Autodesk Inventor part; units mm, degrees
(part 2 of 2)
sketch "Sketch18" plane through (0, 3, 0) normal (0, 1, 0) x (1, 0, 0)
  line L0 (-26.0093, -14.7158) -> (-51.6764, -14.7158)
  line L1 (-51.6764, -14.7158) -> (-51.6764, 17.4536)
  line L2 (-51.6764, 17.4536) -> (-26.0093, 17.4536)
  line L3 (-26.0093, 17.4536) -> (-26.0093, -14.7158)
  line L4 (-61.1366, 28.9911) -> (-74.2787, 28.9911)
  line L5 (-74.2787, 28.9911) -> (-74.2787, 55.1603)
  line L6 (-74.2787, 55.1603) -> (-61.1366, 55.1603)
  line L7 (-61.1366, 55.1603) -> (-61.1366, 28.9911)
  line L8 (-71.136, 57.3703) -> (-87.7064, 57.3703)
  line L9 (-87.7064, 57.3703) -> (-87.7064, 38.1334)
  line L10 (-87.7064, 38.1334) -> (-71.136, 38.1334)
  line L11 (-71.136, 38.1334) -> (-71.136, 57.3703)
  line L12 (-73.3824, 30.8203) -> (-76.7813, 30.8203)
  line L13 (-76.7813, 30.8203) -> (-76.7813, 40.4219)
  line L14 (-76.7813, 40.4219) -> (-73.3824, 40.4219)
  line L15 (-73.3824, 40.4219) -> (-73.3824, 30.8203)
  line L16 (-76.3763, 32.094) -> (-79.4212, 32.094)
  line L17 (-79.4212, 32.094) -> (-79.4212, 39.2374)
  line L18 (-79.4212, 39.2374) -> (-76.3763, 39.2374)
  line L19 (-76.3763, 39.2374) -> (-76.3763, 32.094)
  line L20 (-79.1582, 33.8973) -> (-82.4713, 33.8973)
  line L21 (-82.4713, 33.8973) -> (-82.4713, 38.9159)
  line L22 (-82.4713, 38.9159) -> (-79.1582, 38.9159)
  line L23 (-79.1582, 38.9159) -> (-79.1582, 33.8973)
  line L24 (-82.2476, 35.5049) -> (-85.0994, 35.5049)
  line L25 (-85.0994, 35.5049) -> (-85.0994, 38.3288)
  line L26 (-85.0994, 38.3288) -> (-82.2476, 38.3288)
  line L27 (-82.2476, 38.3288) -> (-82.2476, 35.5049)
  line L28 (-84.8897, 37.1825) -> (-86.2724, 37.1825)
  line L29 (-86.2724, 37.1825) -> (-86.2724, 39.3493)
  line L30 (-86.2724, 39.3493) -> (-84.8897, 39.3493)
  line L31 (-84.8897, 39.3493) -> (-84.8897, 37.1825)
  point P0 (0, 0)
  constraints: 64 end point, 16 parallel, 8 horizontal, 8 perpendicular
extrude "Extrusion18" add sketch "Sketch18" against normal blind 3 contours L4 L5 L12 L15 L10 L11 L6 L7 | L12 L13 L16 L19 L10 L5 | L5 L10 L15 L12 | L11 L10 L15 L14 L5 L6 | L6 L5 L14 L13 L18 L17 L22 L21 L26 L31 L30 L29 L10 L9 L8 L11 | L10 L19 L18 L13 L14 L5 | L5 L14 L15 L10 | L19 L16 L13 L10 | L10 L13 L18 L19 | L16 L17 L20 L23 L10 L13 | L10 L23 L22 L17 L18 L13 | L23 L20 L17 L10 | L10 L17 L22 L23 | L20 L21 L24 L27 L10 L17 | L29 L30 L31 L26 L25 L10 | L10 L27 L26 L21 L22 L17 | L25 L26 L31 L10 | L10 L31 L28 L25 | L27 L24 L21 L10 | L10 L21 L26 L27 | L24 L25 L28 L31 L10 L21 | L31 L26 L21 L10
sketch "Sketch19" plane through (0, 3, 0) normal (0, 1, 0) x (1, 0, 0)
  line L0 (-25.8067, -16.6131) -> (-52.5812, -16.6131)
  line L1 (-52.5812, -16.6131) -> (-52.5812, 17.0969)
  line L2 (-52.5812, 17.0969) -> (-25.8067, 17.0969)
  line L3 (-25.8067, 17.0969) -> (-25.8067, -16.6131)
  line L4 (33.7548, 15.1527) -> (6.613, 15.1527)
  line L5 (6.613, 15.1527) -> (6.613, 48.065)
  line L6 (6.613, 48.065) -> (33.7548, 48.065)
  line L7 (33.7548, 48.065) -> (33.7548, 15.1527)
  line L8 (13.7098, 76.1298) -> (-12.5808, 76.1298)
  line L9 (-12.5808, 76.1298) -> (-12.5808, 99.3558)
  line L10 (-12.5808, 99.3558) -> (13.7098, 99.3558)
  line L11 (13.7098, 99.3558) -> (13.7098, 76.1298)
  line L12 (36.1294, -49.0327) -> (2.2581, -49.0327)
  line L13 (2.2581, -49.0327) -> (2.2581, -15.484)
  line L14 (2.2581, -15.484) -> (36.1294, -15.484)
  line L15 (36.1294, -15.484) -> (36.1294, -49.0327)
  line L16 (13.7098, -98.7106) -> (-12.5808, -98.7106)
  line L17 (-12.5808, -98.7106) -> (-12.5808, -73.7104)
  line L18 (-12.5808, -73.7104) -> (13.7098, -73.7104)
  line L19 (13.7098, -73.7104) -> (13.7098, -98.7106)
  line L20 (86.7795, -30.086) -> (63.0132, -30.086)
  line L21 (63.0132, -30.086) -> (63.0132, -58.4963)
  line L22 (63.0132, -58.4963) -> (86.7795, -58.4963)
  line L23 (86.7795, -58.4963) -> (86.7795, -30.086)
  line L24 (90.7338, 30.2618) -> (63.0132, 30.2618)
  line L25 (63.0132, 30.2618) -> (63.0132, 42.7998)
  line L26 (63.0132, 42.7998) -> (90.7338, 42.7998)
  line L27 (90.7338, 42.7998) -> (90.7338, 30.2618)
  line L28 (87.513, 41.3045) -> (60.8267, 41.3045)
  line L29 (60.8267, 41.3045) -> (60.8267, 56.258)
  line L30 (60.8267, 56.258) -> (87.513, 56.258)
  line L31 (87.513, 56.258) -> (87.513, 41.3045)
  point P0 (0, 0)
  constraints: 64 end point, 16 parallel, 8 horizontal, 8 perpendicular, 3 point on line
extrude "Extrusion19" add sketch "Sketch19" against normal blind 3
sketch "Sketch20" plane through (0, 3, 0) normal (0, 1, 0) x (1, 0, 0)
  line L0 (-88.182, -39.8912) -> (-85.4044, -36.6086)
  line L1 (-85.4044, -36.6086) -> (-74.6729, -30.1276)
  line L2 (-74.6729, -30.1276) -> (-71.0115, -29.5805)
  line L3 (-71.0115, -29.5805) -> (-68.3289, -34.0226)
  line L4 (-68.3289, -34.0226) -> (-62.9313, -48.4344)
  line L5 (-62.9313, -48.4344) -> (-68.3289, -53.8736)
  line L6 (-68.3289, -53.8736) -> (-79.5547, -57.3142)
  line L7 (-79.5547, -57.3142) -> (-88.182, -39.8912)
  point P0 (0, 0)
  constraints: 16 end point, 1 perpendicular, 1 point on line
extrude "Extrusion20" add sketch "Sketch20" against normal blind 3
sketch "Sketch21" plane through (0, 3, 0) normal (0, 1, 0) x (1, 0, 0)
  line L0 (0, 0) -> (-34, 0)
  line L1 (-34, 0) -> (-26, 0)
  line L2 (-26, 0) -> (-26, 10)
  line L3 (-26, 10) -> (-42, 10)
  line L4 (-42, 10) -> (-42, -10)
  line L5 (-42, -10) -> (-26, -10)
  line L6 (-26, -10) -> (-26, 0)
  line L7 (0, 0) -> (17, 29.4449)
  line L8 (0, 0) -> (34, 0) construction
  line L9 (17, 29.4449) -> (13, 22.5167)
  line L10 (13, 22.5167) -> (4.3397, 27.5167)
  line L11 (4.3397, 27.5167) -> (12.3397, 41.3731)
  line L12 (12.3397, 41.3731) -> (29.6603, 31.3731)
  line L13 (29.6603, 31.3731) -> (21.6603, 17.5167)
  line L14 (21.6603, 17.5167) -> (13, 22.5167)
  line L15 (0, 0) -> (17, -29.4449)
  line L16 (0, 0) -> (34, 0) construction
  line L17 (17, -29.4449) -> (13, -22.5167)
  line L18 (13, -22.5167) -> (21.6603, -17.5167)
  line L19 (21.6603, -17.5167) -> (29.6603, -31.3731)
  line L20 (29.6603, -31.3731) -> (12.3397, -41.3731)
  line L21 (12.3397, -41.3731) -> (4.3397, -27.5167)
  line L22 (4.3397, -27.5167) -> (13, -22.5167)
  dimension "d187" = 34
  dimension "d188" = 8
  dimension "d189" = 10
  dimension "d190" = 16
  dimension "d191" = 20
  dimension "d192" = 34
  dimension "d193" = 60
  dimension "d194" = 8
  dimension "d195" = 10
  dimension "d196" = 16
  dimension "d197" = 20
  dimension "d198" = 16
  dimension "d199" = 34
  dimension "d200" = 60
  dimension "d201" = 10
  dimension "d202" = 16
  dimension "d203" = 20
  constraints: 46 end point, 13 perpendicular, 6 point on line, 3 horizontal, 2 equal length
  measures "d187" distance of L0.start L0.end
  measures "d188" distance of L0.end L1.end
  measures "d189" distance of L1.end L2.end
  measures "d190" distance of L2.end L3.end
  measures "d191" distance of L3.end L4.end
  measures "d192" distance of L0.start L7.end
  measures "d193" angle of L8 L7
  measures "d194" distance of L7.end L9.end
  measures "d195" distance of L9.end L10.end
  measures "d196" distance of L10.end L11.end
  measures "d197" distance of L11.end L12.end
  measures "d198" distance of L12.end L13.end
  measures "d199" distance of L0.start L15.end
  measures "d200" angle of L15 L16
  measures "d201" distance of L17.end L18.end
  measures "d202" distance of L18.end L19.end
  measures "d203" distance of L19.end L20.end
extrude "Extrusion21" cut sketch "Sketch21" against normal blind 3
sketch "Sketch22" plane through (0, 3, 0) normal (0, 1, 0) x (1, 0, 0)
  line L0 (0, 0) -> (-73.6122, -42.5)
  line L1 (0, 0) -> (85, 0) construction
  line L2 (-73.6122, -42.5) -> (-64.9519, -37.5)
  line L3 (-64.9519, -37.5) -> (-68.9519, -30.5718)
  line L4 (-68.9519, -30.5718) -> (-86.2724, -40.5718)
  line L5 (-86.2724, -40.5718) -> (-78.2724, -54.4282)
  line L6 (-78.2724, -54.4282) -> (-60.9519, -44.4282)
  line L7 (-60.9519, -44.4282) -> (-64.9519, -37.5)
  line L8 (0, 0) -> (-73.6122, 42.5)
  line L9 (0, 0) -> (85, 0) construction
  line L10 (-73.6122, 42.5) -> (-64.9519, 37.5)
  line L11 (-64.9519, 37.5) -> (-68.9519, 30.5718)
  line L12 (-68.9519, 30.5718) -> (-86.2724, 40.5718)
  line L13 (-86.2724, 40.5718) -> (-78.2724, 54.4282)
  line L14 (-78.2724, 54.4282) -> (-60.9519, 44.4282)
  line L15 (-60.9519, 44.4282) -> (-64.9519, 37.5)
  line L16 (0, 0) -> (0, 85)
  line L17 (0, 85) -> (0, 75)
  line L18 (0, 75) -> (-8, 75)
  line L19 (-8, 75) -> (-8, 95)
  line L20 (-8, 95) -> (8, 95)
  line L21 (8, 95) -> (8, 75)
  line L22 (8, 75) -> (0, 75)
  line L23 (0, 0) -> (73.6122, 42.5)
  line L24 (0, 0) -> (85, 0) construction
  line L25 (73.6122, 42.5) -> (64.9519, 37.5)
  line L26 (64.9519, 37.5) -> (60.9519, 44.4282)
  line L27 (60.9519, 44.4282) -> (78.2724, 54.4282)
  line L28 (78.2724, 54.4282) -> (86.2724, 40.5718)
  line L29 (86.2724, 40.5718) -> (68.9519, 30.5718)
  line L30 (64.9519, 37.5) -> (68.9519, 30.5718)
  line L31 (0, 0) -> (73.6122, -42.5)
  line L32 (73.6122, -42.5) -> (77.6122, -35.5718)
  line L33 (77.6122, -35.5718) -> (68.9519, -30.5718)
  line L34 (68.9519, -30.5718) -> (60.9519, -44.4282)
  line L35 (60.9519, -44.4282) -> (78.2724, -54.4282)
  line L36 (78.2724, -54.4282) -> (86.2724, -40.5718)
  line L37 (86.2724, -40.5718) -> (77.6122, -35.5718)
  line L38 (0, 0) -> (0, -85)
  line L39 (0, -85) -> (0, -75)
  line L40 (0, -75) -> (8, -75)
  line L41 (8, -75) -> (8, -95)
  line L42 (8, -95) -> (-8, -95)
  line L43 (-8, -95) -> (-8, -75)
  line L44 (0, -75) -> (-8, -75)
  dimension "d206" = 85
  dimension "d207" = 150
  dimension "d208" = 10
  dimension "d209" = 8
  dimension "d210" = 20
  dimension "d211" = 16
  dimension "d212" = 85
  dimension "d213" = 150
  dimension "d214" = 8
  dimension "d215" = 20
  dimension "d216" = 16
  dimension "d217" = 85
  dimension "d218" = 10
  dimension "d219" = 8
  dimension "d220" = 20
  dimension "d221" = 16
  dimension "d222" = 85
  dimension "d223" = 30
  dimension "d224" = 8
  dimension "d225" = 20
  dimension "d226" = 20
  dimension "d227" = 10
  dimension "d228" = 20
  dimension "d229" = 16
  constraints: 90 end point, 25 point on line, 23 perpendicular, 3 equal length, 3 horizontal, 1 vertical
  measures "d206" distance of L0.start L0.end
  measures "d207" angle of L0 L1
  measures "d208" distance of L0.end L2.end
  measures "d209" distance of L2.end L3.end
  measures "d210" distance of L3.end L4.end
  measures "d211" distance of L4.end L5.end
  measures "d212" distance of L0.start L8.end
  measures "d213" angle of L9 L8
  measures "d214" distance of L10.end L11.end
  measures "d215" distance of L11.end L12.end
  measures "d216" distance of L12.end L13.end
  measures "d217" distance of L0.start L16.end
  measures "d218" distance of L16.end L17.end
  measures "d219" distance of L17.end L18.end
  measures "d220" distance of L18.end L19.end
  measures "d221" distance of L19.end L20.end
  measures "d222" distance of L0.start L23.end
  measures "d223" angle of L24 L23
  measures "d224" distance of L25.end L26.end
  measures "d225" distance of L26.end L27.end
  measures "d226" distance of L34.end L35.end
  measures "d227" distance of L38.end L39.end
  measures "d228" distance of L40.end L41.end
  measures "d229" distance of L41.end L42.end
extrude "Extrusion22" cut sketch "Sketch22" against normal blind 3
sketch "Sketch23" plane through (0, 3, 0) normal (0, 1, 0) x (1, 0, 0)
  point P0 (0, 0)
fillet "Fillet11" radius 2 12 edges at (-8, 1.5, -95) (8, 1.5, -95) (8, 1.5, -75) (-8, 1.5, -75) (-78.2724, 1.5, -54.4282) (-86.2724, 1.5, -40.5718) (-60.9519, 1.5, -44.4282) (-68.9519, 1.5, -30.5718) (-26, 1.5, -10) (-42, 1.5, -10) (-42, 1.5, 10) (-26, 1.5, 10)
fillet "Fillet12" radius 2 12 edges at (4.3397, 1.5, -27.5167) (12.3397, 1.5, -41.3731) (29.6603, 1.5, -31.3731) (21.6603, 1.5, -17.5167) (60.9519, 1.5, -44.4282) (78.2724, 1.5, -54.4282) (86.2724, 1.5, -40.5718) (68.9519, 1.5, -30.5718) (60.9519, 1.5, 44.4282) (68.9519, 1.5, 30.5718) (86.2724, 1.5, 40.5718) (78.2724, 1.5, 54.4282)
fillet "Fillet13" radius 2 8 edges at (29.6603, 1.5, 31.3731) (21.6603, 1.5, 17.5167) (4.3397, 1.5, 27.5167) (12.3397, 1.5, 41.3731) (-8, 1.5, 75) (8, 1.5, 75) (8, 1.5, 95) (-8, 1.5, 95)
fillet "Fillet14" radius 2 4 edges at (-68.9519, 1.5, 30.5718) (-60.9519, 1.5, 44.4282) (-78.2724, 1.5, 54.4282) (-86.2724, 1.5, 40.5718)
sketch "Sketch24" plane through (0, 3, 0) normal (0, 1, 0) x (1, 0, 0)
  line L0 (0, 0) -> (22.5, 38.9711)
  line L1 (14.0718, 40.3731) -> (27.9282, 32.3731) projected
  line L2 (0, 0) -> (45, 0) construction
  line L3 (0, 0) -> (22.5, -38.9711)
  line L4 (14.0718, -40.3731) -> (27.9282, -32.3731) projected
  line L5 (0, 0) -> (45, 0) construction
  line L6 (0, 0) -> (-45, 0)
  circle A0 centre (22.5, 38.9711) radius 1.5
  circle A1 centre (22.5, -38.9711) radius 1.5
  circle A2 centre (-45, 0) radius 1.5
  dimension "d236" = 45
  dimension "d237" = 60
  dimension "d238" = 45
  dimension "d239" = 60
  dimension "d240" = 45
  dimension "d241" = 3
  dimension "d242" = 3
  constraints: 10 end point, 3 centre point, 3 coincident, 3 horizontal, 2 equal length, 2 perpendicular
  measures "d236" distance of L0.start L0.end
  measures "d237" angle of L2 L0
  measures "d238" distance of L0.start L3.end
  measures "d239" angle of L3 L5
  measures "d240" distance of L0.start L6.end
  measures "d241" diameter of A0
  measures "d242" diameter of A2
extrude "Extrusion23" cut sketch "Sketch24" against normal blind 3
sketch "Sketch25" plane through (0, 3, 0) normal (0, 1, 0) x (1, 0, 0)
  line L0 (-85.2724, -42.3038) -> (-79.2724, -52.6962) projected
  line L1 (-82.2724, -47.5) -> (-80.7724, -50.0981)
  line L2 (-82.2724, -47.5) -> (-84.8705, -49)
  circle A0 centre (-84.8705, -49) radius 1.5
  line L3 (-61.9519, -42.6962) -> (-67.9519, -32.3038) projected
  line L4 (-64.9519, -37.5) -> (-66.4519, -34.9019)
  line L5 (-66.4519, -34.9019) -> (-64.9519, -37.5)
  line L6 (-64.9519, -37.5) -> (-62.3538, -36)
  circle A1 centre (-62.3538, -36) radius 1.5
  line L7 (-67.9519, 32.3038) -> (-61.9519, 42.6962) projected
  line L8 (-64.9519, 37.5) -> (-63.4519, 40.0981)
  line L9 (-63.4519, 40.0981) -> (-64.9519, 37.5)
  line L10 (-64.9519, 37.5) -> (-62.3538, 36)
  circle A2 centre (-62.3538, 36) radius 1.5
  line L11 (-79.2724, 52.6962) -> (-85.2724, 42.3038) projected
  line L12 (-82.2724, 47.5) -> (-83.7724, 44.9019)
  line L13 (-83.7724, 44.9019) -> (-82.2724, 47.5)
  line L14 (-82.2724, 47.5) -> (-84.8705, 49)
  circle A3 centre (-84.8705, 49) radius 1.5
  line L15 (6, 95) -> (-6, 95) projected
  line L16 (0, 95) -> (0, 98)
  line L17 (-6, 75) -> (6, 75) projected
  line L18 (0, 75) -> (0, 72)
  circle A4 centre (0, 72) radius 1.5
  circle A5 centre (0, 98) radius 1.5
  line L19 (79.2724, 52.6962) -> (85.2724, 42.3038) projected
  line L20 (82.2724, 47.5) -> (83.7724, 44.9019)
  line L21 (83.7724, 44.9019) -> (82.2724, 47.5)
  line L22 (82.2724, 47.5) -> (84.8705, 49)
  line L23 (67.9519, 32.3038) -> (61.9519, 42.6962) projected
  line L24 (64.9519, 37.5) -> (63.4519, 40.0981)
  line L25 (63.4519, 40.0981) -> (64.9519, 37.5)
  line L26 (64.9519, 37.5) -> (62.3538, 36)
  circle A6 centre (62.3538, 36) radius 1.5
  circle A7 centre (84.8705, 49) radius 1.5
  line L27 (85.2724, -42.3038) -> (79.2724, -52.6962) projected
  line L28 (82.2724, -47.5) -> (80.7724, -50.0981)
  line L29 (80.7724, -50.0981) -> (82.2724, -47.5)
  line L30 (82.2724, -47.5) -> (84.8705, -49)
  line L31 (61.9519, -42.6962) -> (67.9519, -32.3038) projected
  line L32 (64.9519, -37.5) -> (62.3538, -36)
  line L33 (64.9519, -37.5) -> (67.9519, -37.5) construction
  circle A8 centre (62.3538, -36) radius 1.5
  circle A9 centre (84.8705, -49) radius 1.5
  line L34 (6, -95) -> (-6, -95) projected
  line L35 (0, -95) -> (0, -98)
  line L36 (-6, -75) -> (6, -75) projected
  line L37 (0, -75) -> (0, -72)
  circle A10 centre (0, -72) radius 1.5
  circle A11 centre (0, -98) radius 1.5
  point P0 (0, 0)
  dimension "d245" = 3
  dimension "d246" = 3
  dimension "d247" = 3
  dimension "d248" = 3
  dimension "d249" = 3
  dimension "d250" = 3
  dimension "d251" = 3
  dimension "d252" = 3
  dimension "d253" = 3
  dimension "d254" = 3
  dimension "d255" = 3
  dimension "d256" = 3
  dimension "d257" = 3
  dimension "d258" = 3
  dimension "d259" = 3
  dimension "d260" = 3
  dimension "d261" = 3
  dimension "d262" = 150
  dimension "d263" = 3
  dimension "d264" = 3
  constraints: 52 end point, 12 centre point, 12 coincident, 12 midpoint, 8 perpendicular, 7 point on line, 6 collinear, 4 vertical, 1 equal length, 1 horizontal
  measures "d245" distance of L1.start L1.end
  measures "d246" distance of L1.start L2.end
  measures "d247" distance of L4.start L4.end
  measures "d248" distance of L4.start L6.end
  measures "d249" distance of L8.start L8.end
  measures "d250" distance of L8.start L10.end
  measures "d251" distance of L12.start L12.end
  measures "d252" distance of L12.start L14.end
  measures "d253" distance of L16.start L16.end
  measures "d254" distance of L18.start L18.end
  measures "d255" distance of L20.start L20.end
  measures "d256" distance of L20.start L22.end
  measures "d257" distance of L24.start L24.end
  measures "d258" distance of L24.start L26.end
  measures "d259" distance of L28.start L28.end
  measures "d260" distance of L28.start L30.end
  measures "d261" distance of L32.start L32.end
  measures "d262" angle of L33 L32
  measures "d263" distance of L35.start L35.end
  measures "d264" distance of L37.start L37.end
extrude "Extrusion24" cut sketch "Sketch25" against normal blind 3
sketch "Sketch26" plane through (0, 3, 0) normal (0, 1, 0) x (1, 0, 0)
  line L0 (22.6603, 19.2487) -> (28.6603, 29.641) projected
  line L1 (25.6603, 24.4449) -> (24.1603, 21.8468)
  line L2 (24.1603, 21.8468) -> (25.6603, 24.4449)
  line L3 (25.6603, 24.4449) -> (28.2583, 22.9449)
  line L4 (11.3397, 39.641) -> (5.3397, 29.2487) projected
  line L5 (8.3397, 34.4449) -> (9.8397, 37.0429)
  line L6 (9.8397, 37.0429) -> (8.3397, 34.4449)
  line L7 (8.3397, 34.4449) -> (5.7417, 35.9449)
  line L8 (28.6603, -29.641) -> (22.6603, -19.2487) projected
  line L9 (25.6603, -24.4449) -> (27.1603, -27.0429)
  line L10 (27.1603, -27.0429) -> (25.6603, -24.4449)
  line L11 (25.6603, -24.4449) -> (28.2583, -22.9449)
  line L12 (5.3397, -29.2487) -> (11.3397, -39.641) projected
  line L13 (8.3397, -34.4449) -> (9.8397, -37.0429)
  line L14 (9.8397, -37.0429) -> (8.3397, -34.4449)
  line L15 (8.3397, -34.4449) -> (5.7417, -35.9449)
  line L16 (-28, 10) -> (-40, 10) projected
  line L17 (-34, 10) -> (-34, 13)
  line L18 (-40, -10) -> (-28, -10) projected
  line L19 (-34, -10) -> (-34, -13)
  circle A0 centre (-34, -13) radius 1.5
  circle A1 centre (-34, 13) radius 1.5
  circle A2 centre (5.7417, 35.9449) radius 1.5
  circle A3 centre (28.2583, 22.9449) radius 1.5
  circle A4 centre (28.2583, -22.9449) radius 1.5
  circle A5 centre (5.7417, -35.9449) radius 1.5
  point P0 (0, 0)
  dimension "d267" = 3
  dimension "d268" = 3
  dimension "d269" = 3
  dimension "d270" = 3
  dimension "d271" = 3
  dimension "d272" = 3
  dimension "d273" = 3
  dimension "d274" = 3
  dimension "d275" = 3
  dimension "d276" = 3
  constraints: 28 end point, 6 centre point, 6 coincident, 6 midpoint, 4 collinear, 4 perpendicular, 4 point on line, 2 vertical
  measures "d267" distance of L1.start L1.end
  measures "d268" distance of L1.start L3.end
  measures "d269" distance of L5.start L5.end
  measures "d270" distance of L5.start L7.end
  measures "d271" distance of L9.start L9.end
  measures "d272" distance of L9.start L11.end
  measures "d273" distance of L13.start L13.end
  measures "d274" distance of L13.start L15.end
  measures "d275" distance of L17.start L17.end
  measures "d276" distance of L19.start L19.end
extrude "Extrusion25" cut sketch "Sketch26" against normal blind 3
sketch "Sketch27" plane through (0, 3, 0) normal (0, 1, 0) x (1, 0, 0)
  line L0 (0, 0) -> (89.2708, -32.4919)
  line L1 (0, 0) -> (95, 0) construction
  line L2 (0, 0) -> (89.2708, 32.4919)
  line L3 (0, 0) -> (95, 0) construction
  line L4 (0, 0) -> (-16.4966, 93.5567)
  line L5 (0, 0) -> (95, 0) construction
  line L6 (0, 0) -> (-72.7742, 61.0648)
  line L7 (0, 0) -> (95, 0) construction
  line L8 (0, 0) -> (-72.7742, -61.0648)
  line L9 (0, 0) -> (95, 0) construction
  line L10 (0, 0) -> (-16.4966, -93.5567)
  line L11 (0, 0) -> (95, 0) construction
  circle A0 centre (89.2708, 32.4919) radius 1.5
  circle A1 centre (89.2708, -32.4919) radius 1.5
  circle A2 centre (-16.4966, -93.5567) radius 1.5
  circle A3 centre (-72.7742, -61.0648) radius 1.5
  circle A4 centre (-72.7742, 61.0648) radius 1.5
  circle A5 centre (-16.4966, 93.5567) radius 1.5
  dimension "d279" = 95
  dimension "d280" = 20
  dimension "d281" = 95
  dimension "d282" = 20
  dimension "d283" = 95
  dimension "d284" = 100
  dimension "d285" = 95
  dimension "d286" = 140
  dimension "d287" = 95
  dimension "d288" = 140
  dimension "d289" = 95
  dimension "d290" = 100
  dimension "d291" = 3
  dimension "d292" = 3
  dimension "d293" = 3
  dimension "d294" = 3
  dimension "d295" = 3
  dimension "d296" = 3
  constraints: 24 end point, 6 centre point, 6 coincident, 6 equal length, 6 horizontal
  measures "d279" distance of L0.start L0.end
  measures "d280" angle of L0 L1
  measures "d281" distance of L0.start L2.end
  measures "d282" angle of L3 L2
  measures "d283" distance of L0.start L4.end
  measures "d284" angle of L5 L4
  measures "d285" distance of L0.start L6.end
  measures "d286" angle of L7 L6
  measures "d287" distance of L0.start L8.end
  measures "d288" angle of L8 L9
  measures "d289" distance of L0.start L10.end
  measures "d290" angle of L10 L11
  measures "d291" diameter of A0
  measures "d292" diameter of A1
  measures "d293" diameter of A2
  measures "d294" diameter of A3
  measures "d295" diameter of A4
  measures "d296" diameter of A5
extrude "Extrusion26" cut sketch "Sketch27" against normal blind 3
sketch "Sketch28" plane through (0, 3, 0) normal (0, 1, 0) x (1, 0, 0)
  line L0 (0, 0) -> (27.5, 47.6314)
  line L1 (0, 0) -> (55, 0) construction
  line L2 (0, 0) -> (27.5, -47.6314)
  line L3 (0, 0) -> (55, 0) construction
  line L4 (27.5, -47.6314) -> (18.8176, -96.8718)
  line L5 (27.5, -47.6314) -> (77.5, -47.6314) construction
  line L6 (27.5, -47.6314) -> (74.4846, -64.7324)
  line L7 (27.5, -47.6314) -> (77.5, -47.6314) construction
  line L8 (27.5, 47.6314) -> (74.4846, 64.7324)
  line L9 (27.5, 47.6314) -> (77.5, 47.6314) construction
  line L10 (27.5, 47.6314) -> (18.8176, 96.8718)
  line L11 (27.5, 47.6314) -> (77.5, 47.6314) construction
  arc A0 (74.4846, 64.7324) -> (18.8176, 96.8718) centre (7.4835, 12.9617) ccw
  arc A1 (18.8176, -96.8718) -> (74.4846, -64.7324) centre (8.917, -15.4447) ccw
  dimension "d299" = 55
  dimension "d300" = 60
  dimension "d301" = 55
  dimension "d302" = 60
  dimension "d303" = 50
  dimension "d304" = 100
  dimension "d305" = 50
  dimension "d306" = 20
  dimension "d307" = 50
  dimension "d308" = 20
  dimension "d309" = 50
  dimension "d310" = 100
  constraints: 24 end point, 6 equal length, 6 horizontal, 4 point on circle, 2 centre point
  measures "d299" distance of L0.start L0.end
  measures "d300" angle of L1 L0
  measures "d301" distance of L0.start L2.end
  measures "d302" angle of L2 L3
  measures "d303" distance of L2.end L4.end
  measures "d304" angle of L4 L5
  measures "d305" distance of L2.end L6.end
  measures "d306" angle of L6 L7
  measures "d307" distance of L0.end L8.end
  measures "d308" angle of L9 L8
  measures "d309" distance of L0.end L10.end
  measures "d310" angle of L11 L10
extrude "Extrusion27" cut sketch "Sketch28" against normal blind 3
fillet "Fillet15" radius 5 6 edges at (74.4846, 1.5, -64.7324) (27.5, 1.5, -47.6314) (18.8176, 1.5, -96.8718) (74.4846, 1.5, 64.7324) (27.5, 1.5, 47.6314) (18.8176, 1.5, 96.8718)
fillet "Fillet16" radius 3 3 edges at (-35.7402, 0, -61.9038) (71.4804, 0, 0) (-35.7402, 0, 61.9038)
sketch "Sketch29" plane through (0, 3, 0) normal (0, 1, 0) x (1, 0, 0)
  point P0 (0, 0)
sketch "Sketch30" plane through (0, 3, 0) normal (0, 1, 0) x (1, 0, 0)
  point P0 (0, 0)
sketch "Sketch31" plane through (0, 3, 0) normal (0, 1, 0) x (1, 0, 0)
  line L0 (-71.8236, -69.7966) -> (-73.6166, -71.539) projected
  line L1 (-72.7201, -70.6678) -> (-70.5687, -68.577)
  line L2 (-70.5687, -68.577) -> (-72.7201, -70.6678)
  line L3 (-72.7201, -70.6678) -> (-74.8109, -68.5163)
  line L4 (-25.1463, -99.5233) -> (-24.5338, -97.0994) projected
  line L5 (-24.84, -98.3114) -> (-24.1051, -95.4028)
  line L6 (-24.1051, -95.4028) -> (-24.84, -98.3114)
  line L7 (-24.84, -98.3114) -> (-21.9314, -99.0463)
  circle A0 centre (-21.9314, -99.0463) radius 1.5
  circle A1 centre (-74.8109, -68.5163) radius 1.5
  point P0 (0, 0)
  dimension "d315" = 3
  dimension "d316" = 3
  dimension "d317" = 3
  dimension "d318" = 3
  constraints: 12 end point, 4 collinear, 2 centre point, 2 coincident, 2 midpoint, 2 perpendicular
  measures "d315" distance of L1.start L1.end
  measures "d316" distance of L1.start L3.end
  measures "d317" distance of L5.start L5.end
  measures "d318" distance of L5.start L7.end
extrude "Extrusion28" cut sketch "Sketch31" against normal blind 3
sketch "Sketch32" plane through (0, 3, 0) normal (0, 1, 0) x (1, 0, 0)
  line L0 (-71.8236, 69.7966) -> (-73.6166, 71.539) projected
  line L1 (-72.7201, 70.6678) -> (-70.5687, 68.577)
  line L2 (-70.5687, 68.577) -> (-72.7201, 70.6678)
  line L3 (-72.7201, 70.6678) -> (-74.8109, 68.5163)
  line L4 (-25.1463, 99.5233) -> (-24.5338, 97.0994) projected
  line L5 (-24.84, 98.3114) -> (-25.5749, 101.2199)
  line L6 (-25.5749, 101.2199) -> (-24.84, 98.3114)
  line L7 (-24.84, 98.3114) -> (-21.9314, 99.0463)
  circle A0 centre (-21.9314, 99.0463) radius 1.5
  circle A1 centre (-74.8109, 68.5163) radius 1.5
  line L8 (96.3574, 27.3028) -> (98.7629, 27.9844) projected
  line L9 (97.5601, 27.6436) -> (100.4465, 28.4614)
  line L10 (100.4465, 28.4614) -> (97.5601, 27.6436)
  line L11 (97.5601, 27.6436) -> (96.7423, 30.5299)
  line L12 (98.7629, -27.9844) -> (96.3574, -27.3028) projected
  line L13 (97.5601, -27.6436) -> (100.4465, -28.4614)
  line L14 (100.4465, -28.4614) -> (97.5601, -27.6436)
  line L15 (97.5601, -27.6436) -> (96.7423, -30.5299)
  circle A2 centre (96.7423, -30.5299) radius 1.5
  circle A3 centre (96.7423, 30.5299) radius 1.5
  point P0 (0, 0)
  dimension "d321" = 3
  dimension "d322" = 3
  dimension "d323" = 3
  dimension "d324" = 3
  dimension "d325" = 3
  dimension "d326" = 3
  dimension "d327" = 3
  dimension "d328" = 3
  constraints: 24 end point, 8 collinear, 4 centre point, 4 coincident, 4 midpoint, 3 perpendicular
  measures "d321" distance of L1.start L1.end
  measures "d322" distance of L1.start L3.end
  measures "d323" distance of L5.start L5.end
  measures "d324" distance of L5.start L7.end
  measures "d325" distance of L9.start L9.end
  measures "d326" distance of L9.start L11.end
  measures "d327" distance of L13.start L13.end
  measures "d328" distance of L13.start L15.end
extrude "Extrusion29" cut sketch "Sketch32" against normal blind 3
sketch "Sketch33" plane through (0, 33, 0) normal (0, 1, 0) x (1, 0, 0)
  line L0 (0, 0) -> (-50.0754, 86.7332)
  arc A0 (-26.8396, 96.4875) -> (-70.1408, 71.4875) centre (0, 0) ccw projected
  line L1 (0, 0) -> (100.1509, 0) construction
  line L2 (-25.1463, 99.5233) -> (-24.5338, 97.0994) projected
  arc A1 (-25.1463, 99.5233) -> (-73.6166, 71.539) centre (0, 0) ccw projected
  arc A2 (-25.1463, 99.5233) -> (-25.1463, 99.5233) centre (0, 0) ccw
  arc A3 (-24.5338, 97.0994) -> (-26.8396, 96.4875) centre (0, 0) ccw projected
  arc A4 (-70.1408, 71.4875) -> (-71.8236, 69.7966) centre (0, 0) ccw projected
  arc A5 (-26.8396, 96.4875) -> (-70.1408, 71.4875) centre (0, 0) ccw
  line L3 (-71.8236, 69.7966) -> (-73.6166, 71.539) projected
  line L4 (-71.8236, 69.7966) -> (-73.6166, 71.539)
  dimension "d331" = 120
  constraints: 6 end point, 3 point on circle, 1 centre point, 1 collinear, 1 concentric, 1 equal length, 1 horizontal, 4 other
  measures "d331" angle of L1 L0
extrude "Extrusion30" cut sketch "Sketch33" against normal blind 30 contours A0 A4 L3 A1 L2 A3
sketch "Sketch34" plane through (0, 33, 0) normal (0, 1, 0) x (1, 0, 0)
  arc A0 (-71.8236, -69.7966) -> (-70.1408, -71.4875) centre (0, 0) ccw projected
  arc A1 (-26.8396, -96.4875) -> (-24.5338, -97.0994) centre (0, 0) ccw projected
  arc A2 (-70.1408, -71.4875) -> (-26.8396, -96.4875) centre (0, 0) ccw
  line L0 (-73.6166, -71.539) -> (-71.8236, -69.7966) projected
  line L1 (-24.5338, -97.0994) -> (-25.1463, -99.5233) projected
  arc A3 (-73.6166, -71.539) -> (-25.1463, -99.5233) centre (0, 0) ccw
  line L2 (98.7629, -27.9844) -> (96.3574, -27.3028) projected
  arc A4 (96.9804, 25) -> (96.3574, 27.3028) centre (0, 0) ccw projected
  arc A5 (96.3574, -27.3028) -> (96.9804, 25) centre (0, 0) ccw
  arc A6 (98.7629, -27.9844) -> (98.7629, 27.9844) centre (0, 0) ccw projected
  arc A7 (98.7629, 27.9844) -> (98.7629, -27.9844) centre (0, 0) ccw
  line L3 (96.3574, 27.3028) -> (98.7629, 27.9844) projected
  line L4 (98.7629, 27.9844) -> (96.3574, 27.3028)
  constraints: 8 point on circle, 4 centre point, 2 end point, 1 collinear
extrude "Extrusion31" cut sketch "Sketch34" against normal blind 30 contours A0 A2 A1 L1 A3 L0 | A6 L2 A5 A4 L3
sketch "Sketch35" plane through (0, 3, 0) normal (0, 1, 0) x (1, 0, 0)
  line L0 (-77, -30.5996) -> (-96.3369, -41.7637) projected
  line L1 (-96.3369, -41.7637) -> (-91.5072, -43.0578)
  line L2 (-96.3369, -41.7637) -> (-91.3369, -41.7637) construction
  circle A0 centre (-91.5072, -43.0578) radius 1.5
  arc A1 (-96.3369, -41.7637) -> (-96.3369, 41.7637) centre (0, 0) ccw projected
  line L3 (-96.3369, 41.7637) -> (-91.5072, 43.0578)
  line L4 (-96.3369, 41.7637) -> (-91.3369, 41.7637) construction
  circle A2 centre (-91.5072, 43.0578) radius 1.5
  line L5 (-77, 30.5996) -> (-77, -30.5996) projected
  line L6 (-77, 0) -> (-72, 0)
  circle A3 centre (-72, 0) radius 1.5
  dimension "d336" = 5
  dimension "d337" = 15
  dimension "d338" = 3
  dimension "d339" = 5
  dimension "d340" = 15
  dimension "d341" = 3
  dimension "d342" = 5
  dimension "d343" = 3
  constraints: 10 end point, 3 centre point, 3 coincident, 3 horizontal, 2 equal length, 1 midpoint
  measures "d336" distance of L0.end L1.end
  measures "d337" angle of L1 L2
  measures "d338" diameter of A0
  measures "d339" distance of L3.start L3.end
  measures "d340" angle of L4 L3
  measures "d341" diameter of A2
  measures "d342" distance of L6.start L6.end
  measures "d343" diameter of A3
extrude "Extrusion32" cut sketch "Sketch35" against normal blind 30
sketch "Sketch36" plane through (0, 3, 0) normal (0, 1, 0) x (1, 0, 0)
  point P0 (0, 0)
  point P1 (-77, -30.5996)
  point P2 (-96.3369, -41.7637)
sketch "Sketch37" plane through (0, 33, 0) normal (0, 1, 0) x (1, 0, 0)
  point P0 (0, 0)
  point P1 (-91.5072, -43.0578)
  point P2 (-91.5072, 43.0578)
sketch "Sketch38" plane through (0, 3, 0) normal (0, 1, 0) x (1, 0, 0)
  circle A0 centre (-91.5072, -43.0578) radius 1.5 projected
  circle A1 centre (-91.5072, -43.0578) radius 1.5
  circle A2 centre (-91.5072, 43.0578) radius 1.5 projected
  circle A3 centre (-91.5072, 43.0578) radius 1.5
  point P0 (0, 0)
  constraints: 2 centre point, 2 coincident
extrude "Extrusion33" add sketch "Sketch38" against normal blind 3
sketch "Sketch39" plane through (0, 3, 0) normal (0, 1, 0) x (1, 0, 0)
  line L0 (-77, -30.5996) -> (-96.3369, -41.7637) projected
  line L1 (-96.3369, -41.7637) -> (-92.0067, -39.2637)
  line L2 (-92.0067, -39.2637) -> (-89.5067, -43.5938)
  arc A0 (-96.3369, -41.7637) -> (-96.3369, 41.7637) centre (0, 0) ccw projected
  line L3 (-96.3369, 41.7637) -> (-92.0067, 39.2637)
  line L4 (-96.3369, 41.7637) -> (-77, 30.5996) projected
  line L5 (-92.0067, 39.2637) -> (-89.5067, 43.5938)
  circle A1 centre (-89.5067, 43.5938) radius 1.5
  circle A2 centre (-89.5067, -43.5938) radius 1.5
  dimension "d349" = 5
  dimension "d350" = 5
  dimension "d351" = 5
  dimension "d352" = 5
  dimension "d353" = 3
  dimension "d354" = 3
  constraints: 8 end point, 2 centre point, 2 coincident, 2 perpendicular, 2 point on line
  measures "d349" distance of L0.end L1.end
  measures "d350" distance of L1.end L2.end
  measures "d351" distance of L3.start L3.end
  measures "d352" distance of L3.end L5.end
  measures "d353" diameter of A1
  measures "d354" diameter of A2
extrude "Extrusion34" cut sketch "Sketch39" against normal blind 3
sketch "Sketch40" plane through (0, 3, 0) normal (0, 1, 0) x (1, 0, 0)
  line L0 (-86.415, 38.1584) -> (-84.8879, 36.7457)
  line L1 (-84.8879, 36.7457) -> (-83.915, 38.3181)
  line L2 (-83.915, 38.3181) -> (-85.6515, 39.3925)
  line L3 (-85.6515, 39.3925) -> (-86.415, 38.1584)
  point P0 (0, 0)
  constraints: 8 end point, 2 perpendicular
extrude "Extrusion35" add sketch "Sketch40" against normal blind 3
sketch "Sketch41" plane through (0, 33, 0) normal (0, 1, 0) x (1, 0, 0)
  line L0 (-77, -30.5996) -> (-96.3369, -41.7637) projected
  line L1 (-77, 30.5996) -> (-77, -30.5996) projected
  line L2 (-96.3369, -41.7637) -> (-77, -30.5996)
  line L3 (-96.3369, 41.7637) -> (-77, 30.5996) projected
  line L4 (-77, -30.5996) -> (-77, 30.5996)
  line L5 (-77, 30.5996) -> (-96.3369, 41.7637)
  arc A0 (-97.5, -38.9711) -> (-97.5, 38.9711) centre (0, 0) ccw projected
  line L6 (-97.5, 38.9711) -> (-80, 28.8675) projected
  line L7 (-80, 28.8675) -> (-97.5, 38.9711)
  line L8 (-80, -28.8675) -> (-97.5, -38.9711) projected
  line L9 (-80, 28.8675) -> (-80, -28.8675)
  line L10 (-80, -28.8675) -> (-97.5, -38.9711)
  constraints: 12 end point, 2 collinear, 2 vertical, 1 point on circle
extrude "Extrusion36" cut sketch "Sketch41" against normal blind 30 contours L0 A0 L8 L9 L6 L3 L1
sketch "Sketch42" plane through (0, 3, 0) normal (0, 1, 0) x (1, 0, 0)
  point P0 (0, 0)
sketch "Sketch43" plane through (0, 3, 0) normal (0, 1, 0) x (1, 0, 0)
  point P0 (0, 0)
body "Solid1"
